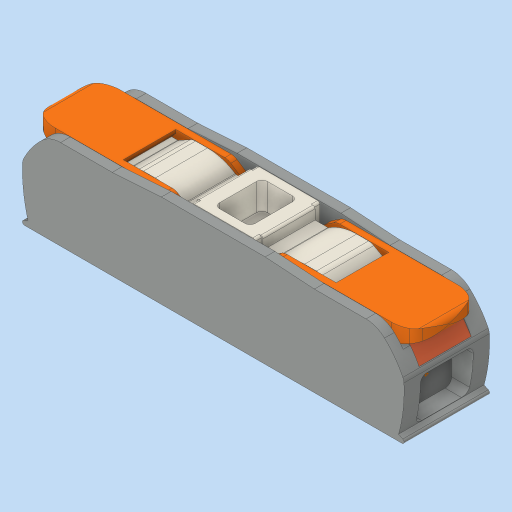
# Autodesk Inventor part: 221-2401
Saved by Autodesk Inventor 2023 (Build 270158000, 158)
## iProperties
Category: PARTsolutions
Company: WAGO
Created: 2023-11-21
Part Number: 221-2401
Material: Generic
Catalog Web Link: www.cadenas.de
Description: 221-2401-Inline splicing connector with lever, for all conductor types, 12 AWG (max.), 2-conductor, transparent housing, white cover, Surrounding air temperature: max 85°C (T85)
Vendor: WAGO
Document SubType Name: Modeling
Designer: psAdmin
Manufacturer: WAGO
Mass: 2.9 g
Surface Area: 21.7408 cm^2
Volume: 2.12144 cm^3
Density: 1 g/cm^3
Appearance: PSOLRGB-142-145-145
Categories: <MemberInstance><Categories><Category DisplayName="" Mnemonic="CABLEANDHARNESS" InternalName="e4a7e005-5e42-4d16-b293-125e7f0d0512"><Category DisplayName="" Mnemonic="CONNECTORS" InternalName="6f634eba-a678-4820-a31d-2c2d5ee6728e"><CategoryParameter DisplayName="" Mnemonic="REFDES" InternalName="c3740e8c-60ab-4d5d-8584-52b73222f2f0"/><Category DisplayName="" Mnemonic="DISCRETEWIRE" InternalName="9a3407de-09b2-4cdb-8c40-9708d5144a28"/></Category></Category></Categories><FamilyTemplate><FamilyTemplateParameters></FamilyTemplateParameters></FamilyTemplate><CategoryParameterMap><ParamToTemplateMap><ParamToTemplate CategoryParameter="//CategoryParameter[@InternalName='c3740e8c-60ab-4d5d-8584-52b73222f2f0']" ConstantValue=""/></ParamToTemplateMap></CategoryParameterMap></MemberInstance>
GlobalPropertyList: <PropertyList/>
PSOL_IDENT_0: {$CADENAS_DATA/23d-libs/wago/pg07/serie221/0221-2401_0999-0962.prj},159 {VTYP=3D},{NB=221-2401},{LIN
PSOL_IDENT_1: A=221-2401},{NN=221-2401},{DATE=14.07.2023 09:43:11},{GEOMDATE=06.04.2023 08:01:51},{VERSION=},{LINE
PSOL_IDENT_2: ID=170},{WBVAR=},{WBNUMERIC=}  {NB=221-2401},{LINA=221-2401},{KT=DUMMY},{BESTNR=221-2401},{BEZEICHNU
PSOL_IDENT_3: NG=Durchgangsverbinder mit Hebel, 4 mm², 32 A, transparent},{INFODE=Info DE},{INFOEN=Info EN},{QUERS
PSOL_IDENT_4: CHNITT1=0.2 - 2.5},{QUERSCHNITT2=18 - 12},{ABISOLIERLAENGE=11},{SPANNUNG=450},{BEMESSSTOSSSPG=4},{VE
PSOL_IDENT_5: RSCHMUTZGRAD=2},{STROM=32},{HOEHE=8.60},{BREITE=7.90},{TIEFE=35.70},{ANZAHLKLEMMSTEL=2},{FARBE=trans
PSOL_IDENT_6: parent},{GEWICHT=2.900},{RGB=0.56,0.57,0.57,0},{ECLASS71=27-14-11-04},{ECLASS81=27-14-11-04},{LINKDE=
PSOL_IDENT_7: http://www.wago.com/de/p/221-2401},{LINKEN=http://www.wago.com/global/p/221-2401},{FILENAME=221-2401
PSOL_IDENT_8: }
NB: 221-2401
NN: 221-2401
NT: Inline splicing connector with lever, for all conductor types, 12 AWG (max.), 2-conductor, transparent housing, white cover, Surrounding air temperature: max 85°C (T85)
NBSYN: $BESTNR.
LINA: 221-2401
CATALOG: WAGO
OFFICIAL_STANDARD_NUMBERS: NO
BESTNR: 221-2401
BEZEICHNUNG: Inline splicing connector with lever, 4 mm², 32 A, transparent
INFODE: Info DE
INFOEN: Info EN
QUERSCHNITT1: 0.2 - 2.5
QUERSCHNITT2: 18 - 12
ABISOLIERLAENGE: 11
SPANNUNG: 450
BEMESSSTOSSSPG: 4
VERSCHMUTZGRAD: 2
STROM: 32
HOEHE: 8.6
BREITE: 7.9
TIEFE: 35.7
ANZAHLKLEMMSTEL: 2
FARBE: transparent
GEWICHT: 2.9
ECLASS71: 27-14-11-04
ECLASS81: 27-14-11-04
SUPPLIER: WAGO
ARTICLENO: 221-2401
BOMINFO: 221-2401
CREATOR: CADENAS GmbH
Title: 221-2401
Author: Cadenas PARTsolutions
Comments: Inline splicing connector with lever, for all conductor types, 12 AWG (max.), 2-conductor, transparent housing, white cover, Surrounding air temperature: max 85°C (T85)
Autodesk Inventor part; units mm, degrees
ref_plane "YZ Plane" through (0, 0, 0) normal (1, 0, 0) x (0, 1, 0)
ref_plane "XZ Plane" through (0, 0, 0) normal (0, 1, 0) x (-1, 0, 0)
ref_plane "XY Plane" through (0, 0, 0) normal (0, 0, 1) x (1, 0, 0)
sketch "Sketch_1" plane through (0, 0, 0) normal (0, 0, 1) x (1, 0, 0)
  arc A0 (-17.6361, 4.9226) -> (-17.1235, 0.5092) centre (-3.74, 4.3) ccw
  arc A1 (-17.1235, 0.5092) -> (-16.45, 0) centre (-16.45, 0.7) ccw
  line L0 (-16.45, 0) -> (16.45, 0)
  arc A2 (16.45, 0) -> (17.1235, 0.5092) centre (16.45, 0.7) ccw
  arc A3 (17.1235, 0.5092) -> (17.6361, 4.9226) centre (3.74, 4.3) ccw
  arc A4 (17.6361, 4.9226) -> (17.5352, 5.3175) centre (16.6371, 4.8778) ccw
  arc A5 (17.5352, 5.3175) -> (15.8408, 7.6182) centre (10.35, 1.8) ccw
  arc A6 (15.8408, 7.6182) -> (14.1249, 8.3) centre (14.1249, 5.8) ccw
  line L1 (14.1249, 8.3) -> (9.35, 8.3)
  line L2 (9.35, 8.3) -> (4.8, 8.6)
  line L3 (4.8, 8.6) -> (-4.8, 8.6)
  line L4 (-4.8, 8.6) -> (-9.35, 8.3)
  line L5 (-9.35, 8.3) -> (-14.1249, 8.3)
  arc A7 (-14.1249, 8.3) -> (-15.8408, 7.6182) centre (-14.1249, 5.8) ccw
  arc A8 (-15.8408, 7.6182) -> (-17.5352, 5.3175) centre (-10.35, 1.8) ccw
  arc A9 (-17.5352, 5.3175) -> (-17.6361, 4.9226) centre (-16.6371, 4.8778) ccw
  constraints: 20 point on circle, 12 end point, 10 centre point
extrude "Extrusion1" add sketch "Sketch_1" along normal blind 7.9
sketch "Sketch_2" plane through (0, 0, 3.95) normal (0, 0, 1) x (1, 0, 0)
  line L0 (-17.65, 6.7) -> (-16.05, 6.7)
  line L1 (-16.05, 6.7) -> (-16.05, 5.4)
  line L2 (-16.05, 5.4) -> (16.05, 5.4)
  line L3 (16.05, 5.4) -> (16.05, 6.7)
  line L4 (16.05, 6.7) -> (17.65, 6.7)
  line L5 (17.65, 6.7) -> (17.65, 8.6)
  line L6 (17.65, 8.6) -> (-17.65, 8.6)
  line L7 (-17.65, 8.6) -> (-17.65, 6.7)
  constraints: 16 end point
extrude "Extrusion2" cut sketch "Sketch_2" along normal mid plane 6.1
sketch "Sketch_3" plane through (0, 0, 3.95) normal (0, 0, 1) x (1, 0, 0)
  line L0 (-17.65, 8.6) -> (-17.65, 5.4)
  line L1 (-17.65, 5.4) -> (17.65, 5.4)
  line L2 (17.65, 5.4) -> (17.65, 8.6)
  line L3 (17.65, 8.6) -> (-17.65, 8.6)
  constraints: 8 end point
extrude "Extrusion3" cut sketch "Sketch_3" along normal mid plane 4.83
sketch "Sketch_4" plane through (0, 0, 3.95) normal (0, 0, 1) x (1, 0, 0)
  line L0 (-17.5, 5.4) -> (17.5, 5.4)
  line L1 (17.5, 5.4) -> (16.5344, 6.8597)
  arc A0 (16.5344, 6.8597) -> (15.25, 7.55) centre (15.25, 6.01) ccw
  line L2 (15.25, 7.55) -> (9.6504, 7.55)
  arc A1 (9.5777, 7.5688) -> (9.6504, 7.55) centre (9.6504, 7.7) ccw
  line L3 (9.5777, 7.5688) -> (8.4848, 8.1746)
  arc A2 (8.4848, 8.1746) -> (8, 8.3) centre (8, 7.3) ccw
  line L4 (8, 8.3) -> (6.9, 8.3)
  arc A3 (6.9, 8.3) -> (4.3234, 7.5249) centre (6.9, 3.63) ccw
  arc A4 (4.2407, 7.5) -> (4.3234, 7.5249) centre (4.2407, 7.65) ccw
  line L5 (4.2407, 7.5) -> (3.05, 7.5)
  line L6 (3.05, 7.5) -> (3.05, 8.4)
  arc A5 (3.05, 8.4) -> (2.85, 8.6) centre (2.85, 8.4) ccw
  line L7 (2.85, 8.6) -> (-2.85, 8.6)
  arc A6 (-2.85, 8.6) -> (-3.05, 8.4) centre (-2.85, 8.4) ccw
  line L8 (-3.05, 8.4) -> (-3.05, 7.5)
  line L9 (-3.05, 7.5) -> (-4.2407, 7.5)
  arc A7 (-4.3234, 7.5249) -> (-4.2407, 7.5) centre (-4.2407, 7.65) ccw
  arc A8 (-4.3234, 7.5249) -> (-6.9, 8.3) centre (-6.9, 3.63) ccw
  line L10 (-6.9, 8.3) -> (-8, 8.3)
  arc A9 (-8, 8.3) -> (-8.4848, 8.1746) centre (-8, 7.3) ccw
  line L11 (-8.4848, 8.1746) -> (-9.5777, 7.5688)
  arc A10 (-9.6504, 7.55) -> (-9.5777, 7.5688) centre (-9.6504, 7.7) ccw
  line L12 (-9.6504, 7.55) -> (-15.25, 7.55)
  arc A11 (-15.25, 7.55) -> (-16.5344, 6.8597) centre (-15.25, 6.01) ccw
  line L13 (-16.5344, 6.8597) -> (-17.5, 5.4)
  constraints: 28 end point, 24 point on circle, 12 centre point
extrude "Extrusion4" add sketch "Sketch_4" along normal mid plane 4.82
sketch "Sketch_5" plane through (0, 0, 3.95) normal (0, 0, 1) x (1, 0, 0)
  line L0 (-2.9, 8.4) -> (-2.9, 6.7)
  line L1 (-2.9, 6.7) -> (2.9, 6.7)
  line L2 (2.9, 6.7) -> (2.9, 8.4)
  arc A0 (2.9, 8.4) -> (2.7, 8.6) centre (2.7, 8.4) ccw
  line L3 (2.7, 8.6) -> (-2.7, 8.6)
  arc A1 (-2.7, 8.6) -> (-2.9, 8.4) centre (-2.7, 8.4) ccw
  constraints: 8 end point, 4 point on circle, 2 centre point
extrude "Extrusion5" add sketch "Sketch_5" along normal mid plane 6
sketch "Sketch_6" plane through (0, 0, 6.98) normal (0, 0, 1) x (1, 0, 0)
  arc A0 (3.9556, 7.591) -> (4.0892, 6.9553) centre (4.15, 7.3) ccw
  line L0 (4.0892, 6.9553) -> (4.65, 6.8564)
  line L1 (4.65, 6.8564) -> (4.65, 3.9)
  arc A1 (4.65, 3.9) -> (8.3007, 2.1391) centre (6.9, 3.9) ccw
  arc A2 (17.4918, 7.2641) -> (8.3007, 2.1391) centre (24.3, -15.75) ccw
  arc A3 (17.4918, 7.2641) -> (17.85, 7.7436) centre (17.35, 7.7436) ccw
  line L2 (17.85, 7.7436) -> (17.85, 7.8)
  arc A4 (17.85, 7.8) -> (17.35, 8.3) centre (17.35, 7.8) ccw
  line L3 (17.35, 8.3) -> (5.32, 8.3)
  arc A5 (5.32, 8.3) -> (4.7644, 8.1315) centre (5.32, 7.3) ccw
  line L4 (4.7644, 8.1315) -> (3.9556, 7.591)
  constraints: 12 point on circle, 10 end point, 6 centre point
extrude "Extrusion6" add sketch "Sketch_6" against normal blind 0.6
sketch "Sketch_7" plane through (0, 0, 6.98) normal (0, 0, 1) x (1, 0, 0)
  arc A0 (-17.85, 7.7436) -> (-17.4918, 7.2641) centre (-17.35, 7.7436) ccw
  arc A1 (-8.3007, 2.1391) -> (-17.4918, 7.2641) centre (-24.3, -15.75) ccw
  arc A2 (-8.3007, 2.1391) -> (-4.65, 3.9) centre (-6.9, 3.9) ccw
  line L0 (-4.65, 3.9) -> (-4.65, 6.8564)
  line L1 (-4.65, 6.8564) -> (-4.0892, 6.9553)
  arc A3 (-4.0892, 6.9553) -> (-3.9556, 7.591) centre (-4.15, 7.3) ccw
  line L2 (-3.9556, 7.591) -> (-4.7644, 8.1315)
  arc A4 (-4.7644, 8.1315) -> (-5.32, 8.3) centre (-5.32, 7.3) ccw
  line L3 (-5.32, 8.3) -> (-17.35, 8.3)
  arc A5 (-17.35, 8.3) -> (-17.85, 7.8) centre (-17.35, 7.8) ccw
  line L4 (-17.85, 7.8) -> (-17.85, 7.7436)
  constraints: 12 point on circle, 10 end point, 6 centre point
extrude "Extrusion7" add sketch "Sketch_7" against normal blind 0.6
sketch "Sketch_8" plane through (0, 0, 0.92) normal (0, 0, 1) x (1, 0, 0)
  arc A0 (3.9556, 7.591) -> (4.0892, 6.9553) centre (4.15, 7.3) ccw
  line L0 (4.0892, 6.9553) -> (4.65, 6.8564)
  line L1 (4.65, 6.8564) -> (4.65, 3.9)
  arc A1 (4.65, 3.9) -> (8.3007, 2.1391) centre (6.9, 3.9) ccw
  arc A2 (17.4918, 7.2641) -> (8.3007, 2.1391) centre (24.3, -15.75) ccw
  arc A3 (17.4918, 7.2641) -> (17.85, 7.7436) centre (17.35, 7.7436) ccw
  line L2 (17.85, 7.7436) -> (17.85, 7.8)
  arc A4 (17.85, 7.8) -> (17.35, 8.3) centre (17.35, 7.8) ccw
  line L3 (17.35, 8.3) -> (5.32, 8.3)
  arc A5 (5.32, 8.3) -> (4.7644, 8.1315) centre (5.32, 7.3) ccw
  line L4 (4.7644, 8.1315) -> (3.9556, 7.591)
  constraints: 12 point on circle, 10 end point, 6 centre point
extrude "Extrusion8" add sketch "Sketch_8" along normal blind 0.6
sketch "Sketch_9" plane through (0, 0, 0.92) normal (0, 0, 1) x (1, 0, 0)
  arc A0 (-17.85, 7.7436) -> (-17.4918, 7.2641) centre (-17.35, 7.7436) ccw
  arc A1 (-8.3007, 2.1391) -> (-17.4918, 7.2641) centre (-24.3, -15.75) ccw
  arc A2 (-8.3007, 2.1391) -> (-4.65, 3.9) centre (-6.9, 3.9) ccw
  line L0 (-4.65, 3.9) -> (-4.65, 6.8564)
  line L1 (-4.65, 6.8564) -> (-4.0892, 6.9553)
  arc A3 (-4.0892, 6.9553) -> (-3.9556, 7.591) centre (-4.15, 7.3) ccw
  line L2 (-3.9556, 7.591) -> (-4.7644, 8.1315)
  arc A4 (-4.7644, 8.1315) -> (-5.32, 8.3) centre (-5.32, 7.3) ccw
  line L3 (-5.32, 8.3) -> (-17.35, 8.3)
  arc A5 (-17.35, 8.3) -> (-17.85, 7.8) centre (-17.35, 7.8) ccw
  line L4 (-17.85, 7.8) -> (-17.85, 7.7436)
  constraints: 12 point on circle, 10 end point, 6 centre point
extrude "Extrusion9" add sketch "Sketch_9" along normal blind 0.6
sketch "Sketch_10" plane through (0, 0, 3.95) normal (0, 0, 1) x (1, 0, 0)
  line L0 (9.85, 8) -> (10.15, 7.62)
  line L1 (10.15, 7.62) -> (15.25, 7.62)
  arc A0 (16.1964, 7.3216) -> (15.25, 7.62) centre (15.25, 5.97) ccw
  line L2 (16.1964, 7.3216) -> (16.4502, 7.1439)
  arc A1 (16.4502, 7.1439) -> (16.8913, 7.0779) centre (16.737, 7.5535) ccw
  arc A2 (17.4918, 7.2641) -> (16.8913, 7.0779) centre (24.3, -15.75) ccw
  arc A3 (17.4918, 7.2641) -> (17.85, 7.7436) centre (17.35, 7.7436) ccw
  line L3 (17.85, 7.7436) -> (17.85, 7.8)
  arc A4 (17.85, 7.8) -> (17.35, 8.3) centre (17.35, 7.8) ccw
  line L4 (17.35, 8.3) -> (9.85, 8.3)
  line L5 (9.85, 8.3) -> (9.85, 8)
  constraints: 12 end point, 10 point on circle, 5 centre point
extrude "Extrusion10" add sketch "Sketch_10" along normal mid plane 4.86
sketch "Sketch_11" plane through (0, 0, 3.95) normal (0, 0, 1) x (1, 0, 0)
  arc A0 (-17.85, 7.7436) -> (-17.4918, 7.2641) centre (-17.35, 7.7436) ccw
  arc A1 (-16.8913, 7.0779) -> (-17.4918, 7.2641) centre (-24.3, -15.75) ccw
  arc A2 (-16.8913, 7.0779) -> (-16.4502, 7.1439) centre (-16.737, 7.5535) ccw
  line L0 (-16.4502, 7.1439) -> (-16.1964, 7.3216)
  arc A3 (-15.25, 7.62) -> (-16.1964, 7.3216) centre (-15.25, 5.97) ccw
  line L1 (-15.25, 7.62) -> (-10.15, 7.62)
  line L2 (-10.15, 7.62) -> (-9.85, 8)
  line L3 (-9.85, 8) -> (-9.85, 8.3)
  line L4 (-9.85, 8.3) -> (-17.35, 8.3)
  arc A4 (-17.35, 8.3) -> (-17.85, 7.8) centre (-17.35, 7.8) ccw
  line L5 (-17.85, 7.8) -> (-17.85, 7.7436)
  constraints: 12 end point, 10 point on circle, 5 centre point
extrude "Extrusion11" add sketch "Sketch_11" along normal mid plane 4.86
sketch "Sketch_12" plane through (0, 8.3, 0) normal (0, 1, 0) x (1, 0, 0)
  line L0 (15.55, -6.98) -> (15.55, -7)
  line L1 (15.55, -7) -> (18.35, -7)
  line L2 (18.35, -7) -> (18.35, -0.9)
  line L3 (18.35, -0.9) -> (15.55, -0.9)
  line L4 (15.55, -0.9) -> (15.55, -0.92)
  arc A0 (16.9042, -1.243) -> (15.55, -0.92) centre (15.55, -3.92) ccw
  arc A1 (17.4907, -1.9048) -> (16.9042, -1.243) centre (16.3625, -2.3138) ccw
  arc A2 (17.4907, -5.9952) -> (17.4907, -1.9048) centre (11.85, -3.95) ccw
  arc A3 (16.9042, -6.657) -> (17.4907, -5.9952) centre (16.3625, -5.5862) ccw
  arc A4 (15.55, -6.98) -> (16.9042, -6.657) centre (15.55, -3.98) ccw
  constraints: 10 end point, 10 point on circle, 5 centre point
extrude "Extrusion12" cut sketch "Sketch_12" against normal blind 1.6
sketch "Sketch_13" plane through (0, 8.3, 0) normal (0, 1, 0) x (1, 0, 0)
  line L0 (-18.35, -7) -> (-15.55, -7)
  line L1 (-15.55, -7) -> (-15.55, -6.98)
  arc A0 (-16.9042, -6.657) -> (-15.55, -6.98) centre (-15.55, -3.98) ccw
  arc A1 (-17.4907, -5.9952) -> (-16.9042, -6.657) centre (-16.3625, -5.5862) ccw
  arc A2 (-17.4907, -1.9048) -> (-17.4907, -5.9952) centre (-11.85, -3.95) ccw
  arc A3 (-16.9042, -1.243) -> (-17.4907, -1.9048) centre (-16.3625, -2.3138) ccw
  arc A4 (-15.55, -0.92) -> (-16.9042, -1.243) centre (-15.55, -3.92) ccw
  line L2 (-15.55, -0.92) -> (-15.55, -0.9)
  line L3 (-15.55, -0.9) -> (-18.35, -0.9)
  line L4 (-18.35, -0.9) -> (-18.35, -7)
  constraints: 10 end point, 10 point on circle, 5 centre point
extrude "Extrusion13" cut sketch "Sketch_13" against normal blind 1.6
sketch "Sketch_14" plane through (0, 8.6, 0) normal (0, 1, 0) x (1, 0, 0)
  arc A0 (-1.65, -5.65) -> (-1.15, -6.15) centre (-1.15, -5.65) ccw
  line L0 (-1.15, -6.15) -> (1.15, -6.15)
  arc A1 (1.15, -6.15) -> (1.65, -5.65) centre (1.15, -5.65) ccw
  line L1 (1.65, -5.65) -> (1.65, -2.25)
  arc A2 (1.65, -2.25) -> (1.15, -1.75) centre (1.15, -2.25) ccw
  line L2 (1.15, -1.75) -> (-1.15, -1.75)
  arc A3 (-1.15, -1.75) -> (-1.65, -2.25) centre (-1.15, -2.25) ccw
  line L3 (-1.65, -2.25) -> (-1.65, -5.65)
  constraints: 8 end point, 8 point on circle, 4 centre point
extrude "Extrusion14" cut sketch "Sketch_14" along normal mid plane 5
sketch "Sketch_15" plane through (17.65, 0, 0) normal (1, 0, 0) x (0, 0, -1)
  line L0 (-6.395, 4.1) -> (-6.395, 1.22)
  arc A0 (-6.395, 1.22) -> (-5.795, 0.62) centre (-5.795, 1.22) ccw
  line L1 (-5.795, 0.62) -> (-2.105, 0.62)
  arc A1 (-2.105, 0.62) -> (-1.505, 1.22) centre (-2.105, 1.22) ccw
  line L2 (-1.505, 1.22) -> (-1.505, 4.1)
  arc A2 (-1.505, 4.1) -> (-2.105, 4.7) centre (-2.105, 4.1) ccw
  line L3 (-2.105, 4.7) -> (-5.795, 4.7)
  arc A3 (-5.795, 4.7) -> (-6.395, 4.1) centre (-5.795, 4.1) ccw
  constraints: 8 end point, 8 point on circle, 4 centre point
extrude "Extrusion15" cut sketch "Sketch_15" against normal blind 2
sketch "Sketch_16" plane through (-17.65, 0, 0) normal (1, 0, 0) x (0, 0, -1)
  line L0 (-6.395, 4.1) -> (-6.395, 1.22)
  arc A0 (-6.395, 1.22) -> (-5.795, 0.62) centre (-5.795, 1.22) ccw
  line L1 (-5.795, 0.62) -> (-2.105, 0.62)
  arc A1 (-2.105, 0.62) -> (-1.505, 1.22) centre (-2.105, 1.22) ccw
  line L2 (-1.505, 1.22) -> (-1.505, 4.1)
  arc A2 (-1.505, 4.1) -> (-2.105, 4.7) centre (-2.105, 4.1) ccw
  line L3 (-2.105, 4.7) -> (-5.795, 4.7)
  arc A3 (-5.795, 4.7) -> (-6.395, 4.1) centre (-5.795, 4.1) ccw
  constraints: 8 end point, 8 point on circle, 4 centre point
extrude "Extrusion16" cut sketch "Sketch_16" along normal blind 2
sketch "Sketch_17" plane through (0, 0, 3.95) normal (0, 0, 1) x (1, 0, 0)
  arc A0 (-17.5345, 0.3813) -> (-17.45, 0) centre (-17.45, 0.2) ccw
  line L0 (-17.45, 0) -> (17.45, 0)
  arc A1 (17.45, 0) -> (17.5345, 0.3813) centre (17.45, 0.2) ccw
  line L1 (17.5345, 0.3813) -> (17.0225, 0.62)
  line L2 (17.0225, 0.62) -> (-17.0225, 0.62)
  line L3 (-17.0225, 0.62) -> (-17.5345, 0.3813)
  constraints: 8 end point, 4 point on circle, 2 centre point
extrude "Extrusion17" add sketch "Sketch_17" along normal mid plane 7.9
sketch "Sketch18" plane through (15.65, 0, 0) normal (1, 0, 0) x (0, 0, -1)
  line L0 (-6.395, 4.1) -> (-6.395, 1.22) projected
  line L1 (-6.395, 2.66) -> (-1.505, 2.66) construction
  line L2 (-1.505, 1.22) -> (-1.505, 4.1) projected
  point P0 (0, 0)
  point P1 (-3.95, 2.66)
  constraints: 3 midpoint, 2 end point
sketch "Sketch19" plane through (-15.65, 0, 0) normal (-1, 0, 0) x (0, 0, 1)
  line L0 (1.505, 1.22) -> (1.505, 4.1) projected
  line L1 (1.505, 2.66) -> (6.395, 2.66) construction
  line L2 (6.395, 4.1) -> (6.395, 1.22) projected
  point P0 (0, 0)
  point P1 (3.95, 2.66)
  constraints: 3 midpoint, 2 end point
body "Solid1"
